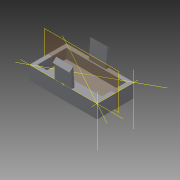
# Autodesk Inventor part: ptt-button
Saved by Autodesk Inventor 2015 (Build 190159000, 159)
## iProperties
Created: 2014-06-24
Part Number: ptt-button
Material: Generic
Document SubType Name: Modeling
Designer: bovine
Density: 1 g/cm^3
Appearance: Default
Author: bovine
Autodesk Inventor part; units mm, degrees
ref_plane "YZ Plane" through (0, 0, 0) normal (1, 0, 0) x (0, 1, 0)
ref_plane "XZ Plane" through (0, 0, 0) normal (0, 1, 0) x (-1, 0, 0)
ref_plane "XY Plane" through (0, 0, 0) normal (0, 0, 1) x (1, 0, 0)
sketch "Sketch1" plane through (0, 0, 0) normal (0, 1, 0) x (-1, 0, 0)
  line L0 (4.6963, 4.4378) -> (-25.5297, 4.4378)
  line L1 (-25.5297, 4.4378) -> (-25.5297, -12.0722)
  line L2 (-25.5297, -12.0722) -> (4.6963, -12.0722)
  line L3 (4.6963, -12.0722) -> (4.6963, 4.4378)
  point P0 (0, 0)
  dimension "d0" = 30.226
  dimension "d1" = 16.51
  constraints: 8 end point, 2 parallel, 1 horizontal, 1 perpendicular
  measures "d0" distance of L2.end L1.end
  measures "d1" distance of L1.end L0.end
extrude "Extrusion1" add sketch "Sketch1" along normal blind 6.096
shell "Shell1" thickness 1.778 removed faces 1 at (15.4543, 6.096, -1.0655)
sketch "Sketch2" plane through (25.5297, 0, 4.4378) normal (1, 0, 0) x (0, 0, -1)
  line L0 (0, -1.7234) -> (-0.5693, -10.1054)
  line L1 (0, -1.7234) -> (8.382, -1.7234) construction
  line L2 (-0.5693, -10.1054) -> (0.7515, -10.1054)
  line L3 (0.7515, -10.1054) -> (0.7515, -3.2474)
  line L4 (0.7515, -3.2474) -> (1.6405, -3.2474)
  line L5 (1.6405, -3.2474) -> (0, -1.7234)
  point P0 (4.4378, 0)
  dimension "d5" = 8.4013
  dimension "d6" = 93.886
  dimension "d7" = 1.3208
  dimension "d8" = 6.858
  dimension "d9" = 0.889
  constraints: 12 end point, 2 perpendicular, 1 horizontal
  measures "d5" distance of L0.start L0.end
  measures "d6" angle of L0 L1
  measures "d7" distance of L0.end L2.end
  measures "d8" distance of L2.end L3.end
  measures "d9" distance of L3.end L4.end
extrude "Extrusion3" add sketch "Sketch2" along normal blind 7.62 separate body
move or copy body "Move Body5" bodies to move or copy 2 copy no translate (-18.923, 16.2052, -15.8496)
ref_plane "Work Plane1" through (-4.6963, 0, -3.8172) normal (0, 0, 1) x (1, 0, 0)
mirror "Mirror1" about plane through (-4.6963, 0, -3.8172) normal (0, 0, 1) bodies 2
combine bodies "Combine1" operation type add bodies to combine 2 1
